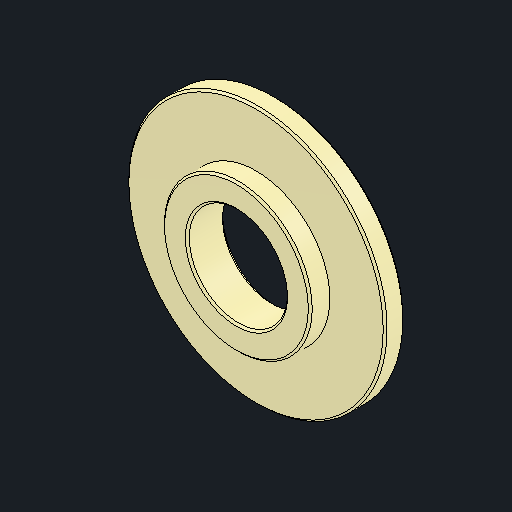
# Autodesk Inventor part: Mesh-mounting-help
Saved by Autodesk Inventor 2025 (Build 290162000, 162)
## iProperties
Created: 2024-07-02
Part Number: Mesh-mounting-help
Material: Nylon 6/6
Document SubType Name: Modeling
Designer: kuzmin
Density: 1.13 g/cm^3
Appearance: Nylon 6
Author: kuzmin
Autodesk Inventor part; units mm, degrees
ref_plane "YZ Plane" through (0, 0, 0) normal (1, 0, 0) x (0, 1, 0)
ref_plane "XZ Plane" through (0, 0, 0) normal (0, 1, 0) x (-1, 0, 0)
ref_plane "XY Plane" through (0, 0, 0) normal (0, 0, 1) x (1, 0, 0)
sketch "Sketch1" plane through (0, 0, 0) normal (0, 1, 0) x (-1, 0, 0)
  line L0 (0, 0) -> (0, 10)
  line L1 (0, 10) -> (18.8, 10)
  line L2 (18.8, 10) -> (18.8, 5)
  line L3 (18.8, 5) -> (32.9, 5)
  line L4 (32.9, 5) -> (32.9, 0)
  line L5 (32.9, 0) -> (0, 0)
  dimension "d0" = 65.8
  dimension "d1" = 37.6
  dimension "d2" = 5
  dimension "d3" = 5
  constraints: 12 end point, 5 perpendicular, 1 vertical
  measures "d0" diameter of L4 L0
  measures "d1" diameter of L2 L0
  measures "d2" distance of L1.end L2.end
  measures "d3" distance of L3.end L4.end
revolve "Revolution1" add sketch "Sketch1" angle 360 about axis through (0, 0, 0) along (0, 0, 1)
hole "Hole1" at (0, 0, 0) direction (0, 0, 1) diameter 25 end through all
chamfer "Chamfer1" distance 0.5 angle 45 4 edges at (32.9, 0, 0) (18.8, 0, 10) (32.9, 0, 5) (0, -12.5, 10)
chamfer "Chamfer2" distance 1 angle 45 1 edges at (0, -12.5, 0)
body "Solid1"
